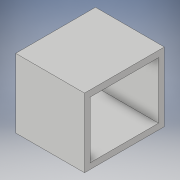
# Autodesk Inventor part: OUTER BODY-2
Saved by Autodesk Inventor 2019 (Build 230136000, 136)
## iProperties
Created: 2019-12-08
Part Number: OUTER BODY-2
Material: Generic
Document SubType Name: Modeling
Designer: HP
Density: 1 g/cm^3
Appearance: Default
Author: HP
Autodesk Inventor part; units mm, degrees
ref_plane "YZ Plane" through (0, 0, 0) normal (1, 0, 0) x (0, 1, 0)
ref_plane "XZ Plane" through (0, 0, 0) normal (0, 1, 0) x (-1, 0, 0)
ref_plane "XY Plane" through (0, 0, 0) normal (0, 0, 1) x (1, 0, 0)
sketch "Sketch1" plane through (0, 0, 0) normal (0, 0, 1) x (1, 0, 0)
  line L0 (0, 0) -> (10.9532, 0)
  line L1 (10.9532, 0) -> (10.9532, 10.9749)
  line L2 (10.9532, 10.9749) -> (0, 10.9749)
  line L3 (0, 10.9749) -> (0, 0)
  constraints: 8 end point, 2 parallel, 1 horizontal, 1 perpendicular
extrude "Extrusion1" add sketch "Sketch1" along normal blind 12.7
sketch "Sketch2" plane through (10.9532, 0, 0) normal (1, 0, 0) x (0, 0, -1)
  line L0 (-11.8225, 9.9752) -> (-0.9128, 9.9752)
  line L1 (-0.9128, 9.9752) -> (-0.9128, 0.9345)
  line L2 (-0.9128, 0.9345) -> (-11.8225, 0.9345)
  line L3 (-11.8225, 0.9345) -> (-11.8225, 9.9752)
  point P0 (0, 0)
  constraints: 8 end point, 2 parallel, 1 horizontal, 1 perpendicular
extrude "Extrusion2" cut sketch "Sketch2" against normal blind 10.16
body "Solid1"
